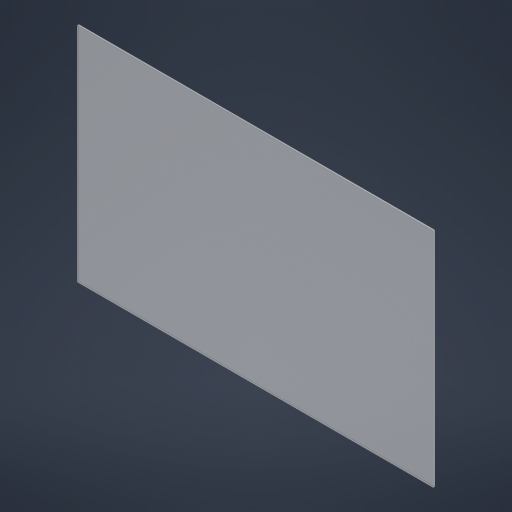
# Autodesk Inventor part: ElectricalPanel
Saved by Autodesk Inventor 2023 (Build 270158000, 158)
## iProperties
Created: 2022-04-16
Part Number: ElectricalPanel
Material: Acrylic, Clear
Document SubType Name: Modeling
Designer: timmy
Density: 1.19 g/cm^3
Appearance: Transparent - Clear
Author: timmy
Autodesk Inventor part; units mm, degrees
ref_plane "YZ Plane" through (0, 0, 0) normal (1, 0, 0) x (0, 1, 0)
ref_plane "XZ Plane" through (0, 0, 0) normal (0, 1, 0) x (-1, 0, 0)
ref_plane "XY Plane" through (0, 0, 0) normal (0, 0, 1) x (1, 0, 0)
sketch "Sketch1" plane through (0, 0, 0) normal (0, 0, 1) x (1, 0, 0)
  line L0 (0, 0) -> (329.692, 0)
  line L1 (329.692, 0) -> (329.692, 206.121)
  line L2 (329.692, 206.121) -> (0, 206.121)
  line L3 (0, 206.121) -> (0, 0)
  dimension "d0" = 329.692
  dimension "d1" = 206.121
  constraints: 8 end point, 2 parallel, 1 horizontal, 1 perpendicular
  measures "d0" distance of L2.end L1.end
  measures "d1" distance between parallel lines of L2 L0
extrude "Extrusion1" add sketch "Sketch1" along normal blind 1.5875
body "Solid1"
